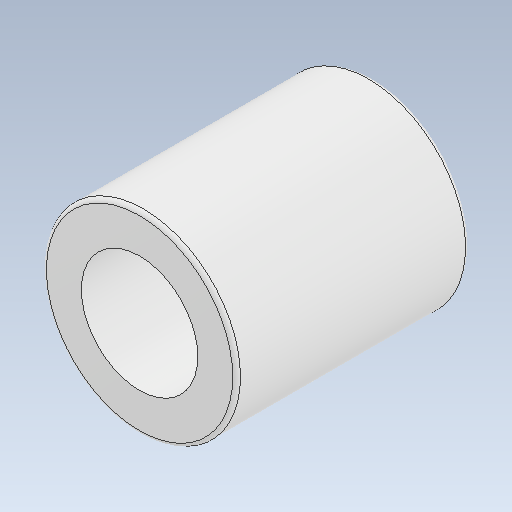
# Autodesk Inventor part: スペーサー中空M6L12樹脂
Saved by Autodesk Inventor 2020.2 (Build 242310000, 310)
## iProperties
Created: 2020-03-18
Part Number: スペーサー中空M6L12樹脂
Material: アセタール樹脂、白
Document SubType Name: Modeling
Designer: aoyam
Density: 1.425 g/cm^3
Appearance: 滑らか - 白
Mass: 0.858778 g
Surface Area: 6.98288 cm^2
Volume: 0.602651 cm^3
Author: aoyam
Autodesk Inventor part; units mm, degrees
ref_plane "YZ Plane" through (0, 0, 0) normal (1, 0, 0) x (0, 1, 0)
ref_plane "XZ Plane" through (0, 0, 0) normal (0, 1, 0) x (-1, 0, 0)
ref_plane "XY Plane" through (0, 0, 0) normal (0, 0, 1) x (1, 0, 0)
sketch "スケッチ1" plane through (0, 0, 0) normal (0, 0, 1) x (1, 0, 0)
  circle A0 centre (0, 0) radius 5
  circle A1 centre (0, 0) radius 3
  dimension "d0" = 10
  dimension "d1" = 6
  constraints: 2 centre point, 2 coincident
  measures "d0" diameter of A0
  measures "d1" diameter of A1
extrude "押し出し1" add sketch "スケッチ1" along normal blind 12
fillet "フィレット1" radius 0.2 2 edges at (-5, 0, 12) (-5, 0, 0)
